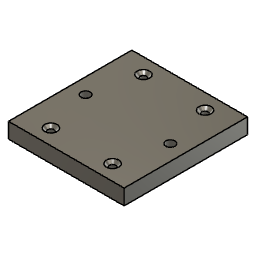
BC carousel holder plate (pls rename) v4 (Autodesk Fusion 360 design; units mm, degrees)
Autodesk Fusion 360 part; units mm, degrees
sketch "Skizze1" plane through (0, 0, 0) normal (0, 1, 0) x (1, 0, 0)
  line L0 (0, 75) -> (0, -65)
  line L1 (0, -50) -> (0, 75)
  line L2 (-85, 0) -> (95, 0)
  line L3 (0, 0) -> (-37.5, 0)
  line L4 (-37.5, 0) -> (-37.5, -25)
  line L5 (-37.5, -25) -> (0, -25)
  line L6 (0, -25) -> (0, 0)
  line L7 (37.5, 0) -> (37.5, -25)
  line L8 (37.5, -25) -> (0, -25)
  line L9 (-37.5, 0) -> (-37.5, 25)
  line L10 (-37.5, 25) -> (0, 25)
  line L11 (37.5, 25) -> (0, 25)
  line L12 (37.5, 0) -> (37.5, 25)
  line L13 (-25.2075, -10.9903) -> (-29.8263, -11.0098)
  line L14 (-29.8263, -11.0098) -> (-32.1188, -15.0195)
  line L15 (-32.1188, -15.0195) -> (-29.7925, -19.0097)
  line L16 (-29.7925, -19.0097) -> (-25.1737, -18.9902)
  line L17 (-25.1737, -18.9902) -> (-22.8812, -14.9805)
  line L18 (-22.8812, -14.9805) -> (-25.2075, -10.9903)
  line L19 (22.8812, -14.9805) -> (25.2075, -10.9903)
  line L20 (25.2075, -10.9903) -> (29.8263, -11.0098)
  line L21 (29.8263, -11.0098) -> (32.1188, -15.0195)
  line L22 (32.1188, -15.0195) -> (29.7925, -19.0097)
  line L23 (29.7925, -19.0097) -> (25.1737, -18.9902)
  line L24 (25.1737, -18.9902) -> (22.8812, -14.9805)
  line L25 (-27.5, -15) -> (27.5, -15) construction
  line L26 (-37.5, -30) -> (-37.5, -55)
  line L27 (-37.5, -30) -> (-37.5, -5)
  line L28 (-37.5, -55) -> (0, -55)
  line L29 (37.5, -55) -> (0, -55)
  line L30 (37.5, -30) -> (37.5, -55)
  line L31 (37.5, -30) -> (37.5, -5)
  point P0 (-27.5, -15)
  point P1 (27.5, -15)
  point P2 (-27.5, -15)
  dimension "d1" = 37.5
  dimension "d2" = 25
  dimension "d7" = 10
  dimension "d8" = 55
  dimension "d9" = 4
  constraint vertical L0
  constraint vertical L1
  constraint horizontal L3
  constraint vertical L4
  constraint horizontal L5
  constraint vertical L6
  constraint coincident L3.start L6.end
  constraint symmetric L1 L3.end L7.start
  constraint symmetric L1 L4.end L7.end
  constraint symmetric L1 L5.end L6.start
  constraint symmetric L2 L3.end L4.start
  constraint symmetric L2 L4.end L9.end
  constraint symmetric L2 L5.end L10.end
  constraint symmetric L2 L7.start L12.start
  constraint symmetric L2 L7.end L11.start
  constraint symmetric L1 P2 P1
  constraint coincident P2 P0
  constraint symmetric L1 L13.start L19.end
  constraint symmetric L1 L13.end L20.end
  constraint symmetric L1 L14.end L21.end
  constraint symmetric L1 L15.end L22.end
  constraint symmetric L1 L16.end L23.end
  constraint symmetric L1 L17.end L19.start
  constraint coincident P1 L25.end
  constraint symmetric L3.end L25 L26.start
  constraint symmetric L4.end L25 L27.end
  constraint symmetric L7.start L25 L30.start
  constraint symmetric L7.end L25 L31.end
  constraint symmetric L9.end L25 L26.end
  constraint symmetric L10.end L25 L28.end
  constraint symmetric L11.start L25 L29.start
  measures "d1" distance of L3.start L3.end
  measures "d2" distance of L3.start L5.end
  measures "d7" distance of L5 P2
  measures "d8" distance of P2 P1
  measures "d9" distance of P2 L18
extrude "Extrusion1" add sketch "Skizze1" along normal blind 10 contours L0 L1 L2 L11 L12 | L0 L1 L2 L3 L9 L10 | L0 L1 L2 L6 L7 L8 L31 | L0 L1 L2 L3 L4 L5 L6 L27 | L0 L1 L8 L29 L30 L31 | L0 L1 L5 L26 L27 L28 | L13 L14 L15 L16 L17 L18 | L19 L20 L21 L22 L23 L24
extrude "Extrusion2" cut sketch "Skizze1" along normal blind 4 contours L13 L14 L15 L16 L17 L18 | L19 L20 L21 L22 L23 L24
ref_plane "Arbeitsebene1" through (0, 10, 15) normal (0, 1, 0) x (0, 0, 1)
sketch "Skizze2" plane through (0, 10, 0) normal (0, 1, 0) x (1, 0, 0)
  line L0 (0, 75) -> (0, -65)
  line L1 (37.5, 25) -> (0, 25)
  line L2 (-27.5, -15) -> (27.5, -15)
  point P0 (-20, 15)
  point P1 (20, 15)
  point P2 (-20, -45)
  point P3 (20, -45)
  dimension "d15" = 40
  dimension "d16" = 10
  constraint symmetric P0 L0 P1
  constraint symmetric P0 L2 P2
  constraint symmetric P1 L2 P3
  measures "d15" distance of P0 P1
  measures "d16" distance of P1 L1
hole "Bohrung1" at (-20, 10, -15) at (20, 10, -15) at (20, 10, 45) at (-20, 10, 45) direction (0, -1, 0) diameter 4.1 end through all countersink diameter 8 countersink angle 90
hole "Bohrung2" at (-27.5, 0, 15) direction (0, 1, 0) diameter 6 depth 12 tip angle 118
mirror "Spiegeln2" about plane through (0, 0, 0) normal (1, 0, 0) of "Bohrung2"
equation "d1 = ( 75 / 2 ) * 1 mm"
equation "d2 = ( 50 / 2 ) * 1 mm"
